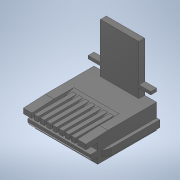
# Autodesk Inventor part: RJ45 Lower Insert
Saved by Autodesk Inventor 2020.1 (Build 241239000, 239)
## iProperties
Created: 2019-12-05
Part Number: RJ45 Lower Insert
Material: PBT Plastic
Document SubType Name: Modeling
Designer: S. Lee
Mass: 1.19075 g
Surface Area: 11.0766 cm^2
Volume: 0.908968 cm^3
Density: 1.31 g/cm^3
Appearance: Smooth - Black
Author: S. Lee
Autodesk Inventor part; units mm, degrees
ref_plane "YZ Plane" through (0, 0, 0) normal (1, 0, 0) x (0, 1, 0)
ref_plane "XZ Plane" through (0, 0, 0) normal (0, 1, 0) x (-1, 0, 0)
ref_plane "XY Plane" through (0, 0, 0) normal (0, 0, 1) x (1, 0, 0)
sketch "Sketch1" plane through (0, 0, 0) normal (0, 0, 1) x (1, 0, 0)
  line L0 (-6.425, 2.5) -> (6.425, 2.5)
  line L1 (6.425, 2.5) -> (6.425, -2.5)
  line L2 (6.425, -2.5) -> (-6.425, -2.5)
  line L3 (-6.425, -2.5) -> (-6.425, 2.5)
  line L4 (-6.425, 2.5) -> (6.425, -2.5) construction
  line L5 (6.425, 2.5) -> (-6.425, -2.5) construction
  line L6 (-6.425, -0.3) -> (-7.06, -0.3)
  line L7 (-7.06, -0.3) -> (-7.06, -1.7)
  line L8 (-7.06, -1.7) -> (-6.425, -1.7)
  line L9 (-6.425, -1.7) -> (-6.425, -0.3)
  line L10 (0, -3.5) -> (0, 3.5) construction
  line L11 (6.425, -0.3) -> (7.06, -0.3)
  line L12 (7.06, -0.3) -> (7.06, -1.7)
  line L13 (7.06, -1.7) -> (6.425, -1.7)
  line L14 (6.425, -1.7) -> (6.425, -0.3)
  line L15 (-4.67, 1.275) -> (-4.22, 1.275)
  line L16 (-4.22, 1.275) -> (-4.22, 0.925)
  line L17 (-4.22, 0.925) -> (-4.67, 0.925)
  line L18 (-4.67, 0.925) -> (-4.67, 1.275)
  line L19 (-2.13, 1.275) -> (-1.68, 1.275)
  line L20 (-2.13, 0.925) -> (-2.13, 1.275)
  line L21 (-1.68, 0.925) -> (-2.13, 0.925)
  line L22 (-1.68, 1.275) -> (-1.68, 0.925)
  line L23 (0.41, 1.275) -> (0.86, 1.275)
  line L24 (0.41, 0.925) -> (0.41, 1.275)
  line L25 (0.86, 0.925) -> (0.41, 0.925)
  line L26 (0.86, 1.275) -> (0.86, 0.925)
  line L27 (2.95, 1.275) -> (3.4, 1.275)
  line L28 (2.95, 0.925) -> (2.95, 1.275)
  line L29 (3.4, 0.925) -> (2.95, 0.925)
  line L30 (3.4, 1.275) -> (3.4, 0.925)
  line L31 (-3.4, -1.265) -> (-2.95, -1.265)
  line L32 (-2.95, -1.265) -> (-2.95, -1.615)
  line L33 (-2.95, -1.615) -> (-3.4, -1.615)
  line L34 (-3.4, -1.615) -> (-3.4, -1.265)
  line L35 (-0.86, -1.615) -> (-0.86, -1.265)
  line L36 (-0.41, -1.615) -> (-0.86, -1.615)
  line L37 (-0.86, -1.265) -> (-0.41, -1.265)
  line L38 (-0.41, -1.265) -> (-0.41, -1.615)
  line L39 (1.68, -1.615) -> (1.68, -1.265)
  line L40 (2.13, -1.615) -> (1.68, -1.615)
  line L41 (1.68, -1.265) -> (2.13, -1.265)
  line L42 (2.13, -1.265) -> (2.13, -1.615)
  line L43 (4.22, -1.615) -> (4.22, -1.265)
  line L44 (4.67, -1.615) -> (4.22, -1.615)
  line L45 (4.22, -1.265) -> (4.67, -1.265)
  line L46 (4.67, -1.265) -> (4.67, -1.615)
  point P0 (0, 0)
  dimension "d0" = 5
  dimension "d1" = 12.85
  dimension "d4" = 1.4
  dimension "d5" = 0.635
  dimension "d6" = 0.8
  dimension "d8" = 1.225
  dimension "d9" = 1.755
  dimension "d10" = 0.35
  dimension "d11" = 0.45
  dimension "d14" = 2.54
  dimension "d23" = 0.35
  dimension "d24" = 0.45
  dimension "d26" = 0.82
  dimension "d27" = 2.19
  dimension "d32" = 2.54
  constraints: 92 end point, 8 parallel, 6 horizontal, 4 perpendicular, 4 symmetric about line, 2 midpoint, 1 point on line, 48 other
  measures "d0" distance of L0.end L1.end
  measures "d1" distance of L0.start L0.end
  measures "d4" distance of L6.end L7.end
  measures "d5" distance of L7.end L8.end
  measures "d6" distance between parallel lines of L2 L8
  measures "d8" distance between parallel lines of L15 L0
  measures "d9" distance between parallel lines of L3 L18
  measures "d10" distance of L15.end L16.end
  measures "d11" distance of L16.end L17.end
  measures "d14" distance of L16.end L21.start
  measures "d23" distance of L32.start L32.end
  measures "d24" distance of L32.end L33.end
  measures "d26" distance between parallel lines of L34 L16
  measures "d27" distance between parallel lines of L31 L17
  measures "d32" distance of L31.start L35.end
extrude "Extrusion1" add sketch "Sketch1" along normal blind 14.5
sketch "Sketch2" plane through (7.06, -1.7, 0) normal (1, 0, 0) x (0, 0, -1)
  line L0 (0, 2.975) -> (-2.4, 2.975)
  line L1 (-2.4, 2.975) -> (-2.4, 1.66)
  line L2 (-2.4, 1.66) -> (-0.9, 1.66)
  line L3 (-0.9, 1.66) -> (-0.9, 1.0475)
  line L4 (-0.9, 1.0475) -> (-1.2536, 0.435)
  line L5 (-1.2536, 0.435) -> (-2.4, 0.435)
  line L6 (-2.4, 0.435) -> (-2.4, -0.8)
  line L7 (0, -0.8) -> (-14.5, -0.8) construction
  line L8 (0, 3.975) -> (-4.5, 4.2)
  line L9 (0, 4.2) -> (-14.5, 4.2) construction
  line L10 (0, 2.975) -> (0, 3.975)
  line L11 (0, 1.4) -> (0, 4.2) construction
  line L12 (-4.5, 4.2) -> (0, 4.2)
  line L13 (0, 4.2) -> (0, 1.4) projected
  line L14 (0, 4.2) -> (0, -0.8)
  line L15 (0, 1.4) -> (0, 0) projected
  line L16 (0, 0) -> (0, -0.8) projected
  line L17 (0, -0.8) -> (-2.4, -0.8)
  dimension "d39" = 4.5
  dimension "d40" = 0.225
  dimension "d41" = 2.4
  dimension "d42" = 1.235
  dimension "d43" = 120
  dimension "d44" = 1.225
  dimension "d45" = 1.315
  dimension "d46" = 1.5
  dimension "d47" = 0.6125
  constraints: 24 end point, 5 collinear, 5 perpendicular, 2 point on line
  measures "d39" distance from line of L11 L8.end
  measures "d40" distance of L9.start L8.start
  measures "d41" distance of L7.start L6.end
  measures "d42" distance of L5.end L6.end
  measures "d43" angle of L4 L5
  measures "d44" distance between parallel lines of L12 L0
  measures "d45" distance of L0.end L1.end
  measures "d46" distance of L1.end L2.end
  measures "d47" distance of L2.end L3.end
extrude "Extrusion2" cut sketch "Sketch2" against normal through all
sketch "Sketch3" plane through (7.06, -1.7, 14.5) normal (1, 0, 0) x (0, 0, -1)
  line L0 (11.4, 1.2) -> (11.4, 0.2)
  line L1 (11.4, 0.2) -> (10, 0)
  line L2 (11.4, 1.2) -> (10, 1.4)
  line L3 (10, 1.4) -> (13.6, 1.4)
  line L4 (13.6, 1.4) -> (13.6, 0)
  line L5 (13.6, 0) -> (10, 0)
  line L6 (13.6, 1.4) -> (0, 1.4) construction
  line L7 (12.1, 0) -> (0, 0) construction
  line L8 (13.6, 1.0475) -> (13.6, 1.4) construction
  line L9 (0, 0) -> (0, 1.4) construction
  dimension "d50" = 1
  dimension "d51" = 11.4
  dimension "d52" = 0.2
  dimension "d53" = 1.4
  dimension "d54" = 1.4
  constraints: 12 end point, 3 collinear, 2 perpendicular, 1 vertical
  measures "d50" distance of L0.start L0.end
  measures "d51" distance between parallel lines of L0 L9
  measures "d52" distance from line of L0.start L3
  measures "d53" horizontal distance of L2.end L0.start
  measures "d54" horizontal distance of L1.end L0.end
extrude "Extrusion3" cut sketch "Sketch3" against normal up to surface (0.635 mm away)
mirror "Mirror1" about plane through (0, 0, 0) normal (1, 0, 0) of "Extrusion3"
chamfer "Chamfer1" distance 1.4 distance2 0.635 1 edges at (7.06, -1, 3.1) measured on face at (7.06, -1, 3.6)
chamfer "Chamfer2" distance 1.4 distance2 0.635 1 edges at (-7.06, -1, 3.1) measured on face at (-7.06, -1, 3.6)
sketch "Sketch4" plane through (0, 0, 0) normal (0, 0, -1) x (-1, 0, 0)
  line L0 (-6.425, 1.275) -> (6.425, 1.275) construction
  line L1 (4.67, 1.275) -> (4.22, 1.275)
  line L2 (4.22, 1.275) -> (4.22, 1.775)
  line L3 (4.22, 1.775) -> (4.67, 1.775)
  line L4 (4.67, 1.775) -> (4.67, 1.275)
  line L5 (4.67, 0.925) -> (4.67, 1.275) construction
  line L6 (3.4, 1.275) -> (2.95, 1.275)
  line L7 (2.95, 1.275) -> (2.95, 1.775)
  line L8 (2.95, 1.775) -> (3.4, 1.775)
  line L9 (3.4, 1.775) -> (3.4, 1.275)
  line L10 (2.13, 1.275) -> (1.68, 1.275)
  line L11 (1.68, 1.275) -> (1.68, 1.775)
  line L12 (1.68, 1.775) -> (2.13, 1.775)
  line L13 (2.13, 1.775) -> (2.13, 1.275)
  line L14 (0.86, 1.275) -> (0.41, 1.275)
  line L15 (0.41, 1.275) -> (0.41, 1.775)
  line L16 (0.41, 1.775) -> (0.86, 1.775)
  line L17 (0.86, 1.775) -> (0.86, 1.275)
  line L18 (-0.41, 1.275) -> (-0.86, 1.275)
  line L19 (-0.86, 1.275) -> (-0.86, 1.775)
  line L20 (-0.86, 1.775) -> (-0.41, 1.775)
  line L21 (-0.41, 1.775) -> (-0.41, 1.275)
  line L22 (-1.68, 1.275) -> (-2.13, 1.275)
  line L23 (-2.13, 1.275) -> (-2.13, 1.775)
  line L24 (-2.13, 1.775) -> (-1.68, 1.775)
  line L25 (-1.68, 1.775) -> (-1.68, 1.275)
  line L26 (-2.95, 1.275) -> (-3.4, 1.275)
  line L27 (-3.4, 1.275) -> (-3.4, 1.775)
  line L28 (-3.4, 1.775) -> (-2.95, 1.775)
  line L29 (-2.95, 1.775) -> (-2.95, 1.275)
  line L30 (-4.22, 1.275) -> (-4.67, 1.275)
  line L31 (-4.67, 1.275) -> (-4.67, 1.775)
  line L32 (-4.67, 1.775) -> (-4.22, 1.775)
  line L33 (-4.22, 1.775) -> (-4.22, 1.275)
  point P0 (0, 0)
  dimension "d63" = 0.45
  dimension "d64" = 0.5
  dimension "d67" = 1.27
  constraints: 64 end point, 2 horizontal, 2 parallel, 1 collinear, 1 perpendicular, 1 point on line, 56 other
  measures "d63" distance of L2.end L3.end
  measures "d64" distance of L1.end L2.end
  measures "d67" distance of L1.start L6.start
extrude "Extrusion4" cut sketch "Sketch4" against normal blind 0.35
sketch "Sketch5" plane through (0, 0, 0) normal (0, 0, -1) x (-1, 0, 0)
  line L0 (4.22, 1.775) -> (4.67, 1.775) construction
  line L1 (2.95, 1.775) -> (3.4, 1.775) construction
  line L2 (1.68, 1.775) -> (2.13, 1.775) construction
  line L3 (0.41, 1.775) -> (0.86, 1.775) construction
  line L4 (-0.86, 1.775) -> (-0.41, 1.775) construction
  line L5 (-3.4, 1.775) -> (-2.95, 1.775) construction
  line L6 (-4.67, 1.775) -> (-4.22, 1.775) construction
  line L7 (-6.425, 2.5) -> (6.425, 2.5) construction
  line L8 (-2.13, 1.775) -> (-1.68, 1.775) construction
  line L9 (-4.67, 1.275) -> (-4.67, 1.775) construction
  line L10 (-6.425, 2.5) -> (6.425, 2.5) projected
  line L11 (-4.67, 1.775) -> (-4.22, 1.775)
  line L12 (-4.22, 1.775) -> (-4.22, 2.5)
  line L13 (-4.22, 2.5) -> (-4.67, 2.5)
  line L14 (-4.67, 2.5) -> (-4.67, 1.775)
  line L15 (-4.22, 1.775) -> (-4.22, 1.275) construction
  line L16 (-2.95, 1.775) -> (-2.95, 2.5)
  line L17 (-3.4, 2.5) -> (-3.4, 1.775)
  line L18 (-2.95, 2.5) -> (-3.4, 2.5)
  line L19 (-3.4, 1.775) -> (-2.95, 1.775)
  line L20 (-1.68, 1.775) -> (-1.68, 2.5)
  line L21 (-2.13, 2.5) -> (-2.13, 1.775)
  line L22 (-1.68, 2.5) -> (-2.13, 2.5)
  line L23 (-2.13, 1.775) -> (-1.68, 1.775)
  line L24 (-0.41, 1.775) -> (-0.41, 2.5)
  line L25 (-0.86, 2.5) -> (-0.86, 1.775)
  line L26 (-0.41, 2.5) -> (-0.86, 2.5)
  line L27 (-0.86, 1.775) -> (-0.41, 1.775)
  line L28 (0.86, 1.775) -> (0.86, 2.5)
  line L29 (0.41, 2.5) -> (0.41, 1.775)
  line L30 (0.86, 2.5) -> (0.41, 2.5)
  line L31 (0.41, 1.775) -> (0.86, 1.775)
  line L32 (2.13, 1.775) -> (2.13, 2.5)
  line L33 (1.68, 2.5) -> (1.68, 1.775)
  line L34 (2.13, 2.5) -> (1.68, 2.5)
  line L35 (1.68, 1.775) -> (2.13, 1.775)
  line L36 (3.4, 1.775) -> (3.4, 2.5)
  line L37 (2.95, 2.5) -> (2.95, 1.775)
  line L38 (3.4, 2.5) -> (2.95, 2.5)
  line L39 (2.95, 1.775) -> (3.4, 1.775)
  line L40 (4.67, 1.775) -> (4.67, 2.5)
  line L41 (4.22, 2.5) -> (4.22, 1.775)
  line L42 (4.67, 2.5) -> (4.22, 2.5)
  line L43 (4.22, 1.775) -> (4.67, 1.775)
  line L44 (-4.67, 2.5) -> (4.67, 2.5)
  line L45 (4.67, 2.5) -> (4.67, 2.275)
  line L46 (4.67, 2.275) -> (-4.67, 2.275)
  line L47 (-4.67, 2.275) -> (-4.67, 2.5)
  point P0 (0, 0)
  point P1 (-4.22, 2.275)
  point P2 (-3.4, 2.275)
  point P3 (-2.95, 2.275)
  point P4 (-2.13, 2.275)
  point P5 (-1.68, 2.275)
  point P6 (-0.86, 2.275)
  point P7 (-0.41, 2.275)
  point P8 (0.41, 2.275)
  point P9 (0.86, 2.275)
  point P10 (1.68, 2.275)
  point P11 (2.13, 2.275)
  point P12 (2.95, 2.275)
  point P13 (3.4, 2.275)
  point P14 (4.22, 2.275)
  dimension "d76" = 1.27
  dimension "d83" = 0.225
  constraints: 72 end point, 4 parallel, 3 horizontal, 2 perpendicular, 2 point on line, 1 collinear, 56 other
  measures "d76" distance of L11.end L16.start
  measures "d83" distance between parallel lines of L7 L46
extrude "Extrusion5" cut sketch "Sketch5" against normal blind 6.5
chamfer "Chamfer3" distance 2.1 distance2 0.725 1 edges at (0, 2.5, 6.5)
sketch "Sketch6" plane through (0, 0, 14.5) normal (0, 0, 1) x (1, 0, 0)
  line L0 (-4.67, 2.5) -> (4.67, 2.5) projected
  line L1 (-3.99, 2.5) -> (3.99, 2.5)
  line L2 (3.99, 2.5) -> (3.99, 12.65)
  line L3 (3.99, 12.65) -> (-3.99, 12.65)
  line L4 (-3.99, 12.65) -> (-3.99, 2.5)
  line L5 (-6.425, 4.975) -> (6.425, 4.975)
  line L6 (6.425, 4.975) -> (6.425, 4.375)
  line L7 (6.425, 4.375) -> (-6.425, 4.375)
  line L8 (-6.425, 4.375) -> (-6.425, 4.975)
  line L9 (0, -4.5055) -> (0, 9.5333) projected
  point P0 (0, 0)
  point P1 (3.99, 4.975)
  point P2 (-3.99, 4.975)
  point P3 (-3.99, 4.375)
  point P4 (3.99, 4.375)
  dimension "d87" = 7.98
  dimension "d88" = 12.85
  dimension "d89" = 0.6
  dimension "d90" = 10.15
  dimension "d91" = 1.875
  constraints: 16 end point, 4 parallel, 2 horizontal, 2 perpendicular, 1 point on line, 2 other
  measures "d87" distance of L2.end L3.end
  measures "d88" distance of L5.start L5.end
  measures "d89" distance of L7.end L5.start
  measures "d90" distance of L3.end L1.start
  measures "d91" distance between parallel lines of L7 L0
extrude "Extrusion6" add sketch "Sketch6" against normal blind 1.2
fillet "Fillet1" radius 0.1 18 edges at (4.445, 1.775, 0.35) (4.445, 1.275, 0.35) (3.175, 1.775, 0.35) (3.175, 1.275, 0.35) (1.905, 1.775, 0.35) (1.905, 1.275, 0.35) (0.635, 1.275, 0.35) (0.635, 1.775, 0.35) (-0.635, 1.775, 0.35) (-0.635, 1.275, 0.35) (-1.905, 1.775, 0.35) (-1.905, 1.275, 0.35) (-3.175, 1.775, 0.35) (-3.175, 1.275, 0.35) (-4.445, 1.775, 0.35) (-4.445, 1.275, 0.35) (-3.99, 12.65, 13.9) (3.99, 12.65, 13.9)
move or copy body "Move Body1" bodies to move or copy 1 copy no rotation origin (0, 0, 0) rotation axis (0, 1, 0) rotation angle 180
move or copy body "Move Body2" bodies to move or copy 1 copy no translate (10, 0, 0)
move or copy body "Move Body3" bodies to move or copy 1 copy no translate (0, 0, 7.25)
move or copy body "Move Body4" bodies to move or copy 1 copy no translate (-10, 0, 0)
body "Solid1"
